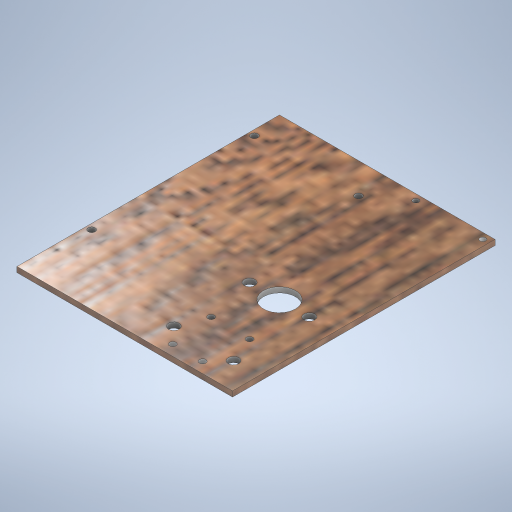
# Autodesk Inventor part: BaseMDF
Saved by Autodesk Inventor 2024 (Build 280153000, 153)
## iProperties
Created: 2024-06-04
Part Number: BaseMDF
Material: Genérico
Document SubType Name: Modeling
Designer: alexa
Density: 1 g/cm^3
Appearance: Valor por defecto
Author: alexa
Autodesk Inventor part; units mm, degrees
ref_plane "YZ Plane" through (0, 0, 0) normal (1, 0, 0) x (0, 1, 0)
ref_plane "XZ Plane" through (0, 0, 0) normal (0, 1, 0) x (-1, 0, 0)
sketch "Sketch1" plane through (0, 0, 0) normal (0, 1, 0) x (-1, 0, 0)
  line L0 (75, 48) -> (75, -75)
  line L1 (75, -75) -> (-26, -75)
  line L2 (-26, -75) -> (-26, 48)
  line L3 (75, 48) -> (-26, 48)
  point P0 (0, 0)
  constraints: 8 end point
extrude "Extrusion1" add sketch "Sketch1" along normal blind 2.5
sketch "Sketch2" plane through (0, 2.5, 0) normal (0, 1, 0) x (1, 0, 0)
  circle A0 centre (0, 0) radius 7.5
  dimension "d4" = 15
  constraints: 1 centre point, 1 coincident
  measures "d4" diameter of A0
extrude "Extrusion2" cut sketch "Sketch2" against normal blind 2.5
ref_plane "Work Plane1" through (0, 0, 48) normal (1, 0, 0) x (0, 0, -1)
sketch "Sketch3" plane through (0, 0, 0) normal (0, -1, 0) x (1, 0, 0)
  circle A0 centre (7, 43) radius 1.5
  line L0 (26, 48) -> (26, -75) projected
  line L1 (-75, 48) -> (26, 48) projected
  circle A1 centre (9, 23) radius 1.5
  point P0 (0, 0)
  dimension "d12" = 3
  dimension "d15" = 19
  dimension "d18" = 3
  dimension "d19" = 17
  dimension "d20" = 25
  dimension "d21" = 5
  constraints: 2 centre point
  measures "d12" diameter of A0
  measures "d15" distance from line of L0 A0.centre
  measures "d18" diameter of A1
  measures "d19" distance from line of L0 A1.centre
  measures "d20" vertical distance of L0.start A1.centre
  measures "d21" vertical distance of A0.centre L0.start
extrude "Extrusion3" cut sketch "Sketch3" against normal blind 2.5
mirror "Mirror1" about plane through (0, 0, 48) normal (1, 0, 0) of "Extrusion3"
sketch "Sketch4" plane through (0, 0, 0) normal (0, -1, 0) x (1, 0, 0)
  line L0 (-75, 48) -> (26, 48) projected
  circle A0 centre (14, 35.5) radius 2.5
  circle A1 centre (14, 0) radius 2.5
  point P0 (0, 0)
  dimension "d24" = 5
  dimension "d28" = 5
  dimension "d29" = 14
  dimension "d30" = 14
  constraints: 2 centre point
  measures "d24" diameter of A0
  measures "d28" diameter of A1
  measures "d29" horizontal distance of point (0, 0) A0.centre
  measures "d30" distance of point (0, 0) A1.centre
extrude "Extrusion4" cut sketch "Sketch4" against normal blind 2.5
mirror "Mirror2" about plane through (0, 0, 48) normal (1, 0, 0) of "Extrusion4"
sketch "Sketch5" plane through (0, 0, 0) normal (0, -1, 0) x (1, 0, 0)
  line L0 (26, 48) -> (26, -75) projected
  circle A0 centre (23.15, -72.15) radius 1.35
  point P0 (0, 0)
  dimension "d33" = 2.7
  constraints: 1 centre point
  measures "d33" diameter of A0
extrude "Extrusion5" cut sketch "Sketch5" against normal blind 2.5
pattern_linear "Rectangular Pattern1" count 2 spacing 31.4 along (-1, 0, 0) of "Extrusion5"
sketch "Sketch6" plane through (0, 0, 0) normal (0, -1, 0) x (1, 0, 0)
  circle A0 centre (-72.4, -60.65) radius 1.65
  point P0 (0, 0)
  point P1 (-75, -75)
  dimension "d41" = 3.3
  constraints: 1 centre point
  measures "d41" diameter of A0
extrude "Extrusion6" cut sketch "Sketch6" against normal blind 2.5
pattern_linear "Rectangular Pattern2" count 2 spacing 48.8 along (1, 0, 0) of "Extrusion6"
pattern_linear "Rectangular Pattern3" count 2 spacing 76.25 along (0, 0, 1) of "Extrusion6"
body "Solid1"
